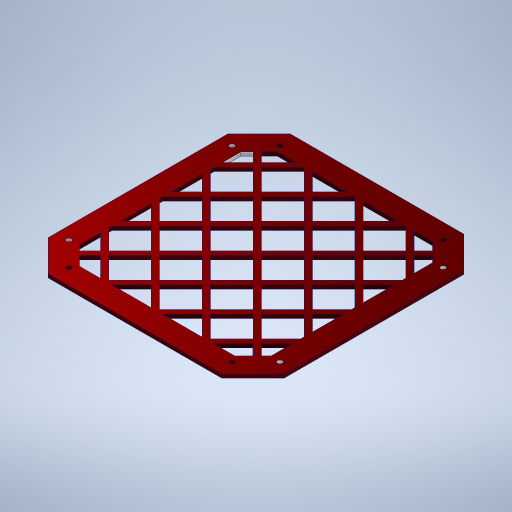
# Autodesk Inventor part: Part2
Saved by Autodesk Inventor 2024.2 (Build 282272000, 272)
## iProperties
Created: 2024-01-05
Part Number: Part2
Material: Aluminum 6061
Document SubType Name: Modeling
Designer: rohan
Density: 2.7 g/cm^3
Appearance: Aluminum - Flat
Author: rohan
Autodesk Inventor part; units mm, degrees
ref_plane "YZ Plane" through (0, 0, 0) normal (1, 0, 0) x (0, 1, 0)
ref_plane "XZ Plane" through (0, 0, 0) normal (0, 1, 0) x (-1, 0, 0)
ref_plane "XY Plane" through (0, 0, 0) normal (0, 0, 1) x (1, 0, 0)
sketch "Sketch4" plane through (0, 0, 0) normal (0, 1, 0) x (-1, 0, 0)
  line L0 (101.6, 104.2289) -> (-101.6, 104.2289)
  line L1 (-101.6, 104.2289) -> (-101.6, -104.2289)
  line L2 (-101.6, -104.2289) -> (101.6, -104.2289)
  line L3 (101.6, -104.2289) -> (101.6, 104.2289)
  line L4 (101.6, 104.2289) -> (-101.6, -104.2289) construction
  line L5 (-101.6, 104.2289) -> (101.6, -104.2289) construction
  point P0 (0, 0)
  dimension "d27" = 203.2
  dimension "d28" = 208.4578
  constraints: 12 end point, 2 midpoint, 2 parallel, 1 horizontal, 1 perpendicular
  measures "d27" distance of L2.end L1.end
  measures "d28" distance of L1.end L0.end
extrude "Extrusion4" add sketch "Sketch4" along normal blind 3.175
sketch "Sketch5" plane through (0, 3.175, 0) normal (0, 1, 0) x (1, 0, 0)
  line L0 (101.6, -104.2289) -> (101.6, 104.2289) projected
  line L1 (101.6, 104.2289) -> (-101.6, 104.2289) projected
  line L2 (-101.6, 104.2289) -> (-101.6, -104.2289) projected
  line L3 (-101.6, -104.2289) -> (101.6, -104.2289) projected
  line L4 (70.2691, 90.8431) -> (-70.2691, 90.8431)
  line L5 (-70.2691, 90.8431) -> (-70.2691, -90.8431)
  line L6 (-70.2691, -90.8431) -> (70.2691, -90.8431)
  line L7 (70.2691, -90.8431) -> (70.2691, 90.8431)
  line L8 (70.2691, 90.8431) -> (-70.2691, -90.8431) construction
  line L9 (-70.2691, 90.8431) -> (70.2691, -90.8431) construction
  circle A0 centre (-70.2691, -90.8431) radius 1.9939
  circle A1 centre (-70.2691, 90.8431) radius 1.9939
  circle A2 centre (70.2691, 90.8431) radius 1.9939
  circle A3 centre (70.2691, -90.8431) radius 1.9939
  point P0 (0, 0)
  dimension "d31" = 203.2
  dimension "d32" = 208.4578
  dimension "d33" = 140.5382
  dimension "d34" = 181.6862
  dimension "d39" = 3.9878
  dimension "d40" = 3.9878
  dimension "d41" = 3.9878
  dimension "d42" = 3.9878
  constraints: 12 end point, 4 centre point, 4 coincident, 2 midpoint, 2 parallel, 1 horizontal, 1 perpendicular
  measures "d31" distance of L2.end L0.start
  measures "d32" distance of L1.end L2.end
  measures "d33" distance of L6.end L5.end
  measures "d34" distance of L5.end L4.end
  measures "d39" diameter of A0
  measures "d40" diameter of A1
  measures "d41" diameter of A2
  measures "d42" diameter of A3
extrude "Extrusion7" cut sketch "Sketch5" against normal blind 26.9875 contours A1 L5 L4 | L4 L5 A1 | A2 L7 L4 | L4 L7 A2 | A0 L6 L5 | L5 L6 A0 | A3 L6 L7 | L7 L6 A3
chamfer "Chamfer1" distance 26.9875 angle 45 1 edges at (101.6, 1.5875, 104.2289)
chamfer "Chamfer2" distance 26.9875 angle 45 3 edges at (101.6, 1.5875, -104.2289) (-101.6, 1.5875, -104.2289) (-101.6, 1.5875, 104.2289)
sketch "Sketch8" plane through (0, 3.175, 0) normal (0, 1, 0) x (1, 0, 0)
  circle A0 centre (70.2691, 90.8431) radius 1.9939 projected
  circle A1 centre (70.2691, -90.8431) radius 1.9939 projected
  circle A2 centre (-70.2691, 90.8431) radius 1.9939 projected
  circle A3 centre (-70.2691, -90.8431) radius 1.9939 projected
  line L0 (-74.6125, -104.2289) -> (-101.6, -77.2414) projected
  line L1 (-74.6125, -104.2289) -> (74.6125, -104.2289) projected
  line L2 (101.6, -77.2414) -> (74.6125, -104.2289) projected
  line L3 (101.6, -77.2414) -> (101.6, 77.2414) projected
  line L4 (74.6125, 104.2289) -> (101.6, 77.2414) projected
  line L5 (74.6125, 104.2289) -> (-74.6125, 104.2289) projected
  line L6 (-101.6, 77.2414) -> (-74.6125, 104.2289) projected
  line L7 (-101.6, 77.2414) -> (-101.6, -77.2414) projected
  line L8 (66.7217, -85.1789) -> (-66.7217, -85.1789)
  line L9 (-66.7217, -85.1789) -> (-82.55, -69.3506)
  line L10 (-82.55, -69.3506) -> (-82.55, 69.3506)
  line L11 (-82.55, 69.3506) -> (-66.7217, 85.1789)
  line L12 (-66.7217, 85.1789) -> (66.7217, 85.1789)
  line L13 (66.7217, 85.1789) -> (82.55, 69.3506)
  line L14 (82.55, 69.3506) -> (82.55, -69.3506)
  line L15 (82.55, -69.3506) -> (66.7217, -85.1789)
  line L16 (82.55, -51.3901) -> (48.7612, -85.1789)
  line L17 (91.8895, -34.8664) -> (32.2375, -94.5184)
  line L18 (85.1946, -41.5613) -> (82.55, -44.2059)
  line L19 (34.1074, -92.6485) -> (41.577, -85.1789)
  line L20 (74.6359, -77.2648) -> (62.9721, -65.601)
  line L21 (69.9776, -12.9546) -> (10.3257, -72.6065)
  line L22 (60.6382, -29.4783) -> (26.8494, -63.2671)
  line L23 (12.1956, -70.7367) -> (19.6652, -63.2671)
  line L24 (63.2827, -19.6495) -> (60.6382, -22.2941)
  line L25 (48.0658, 8.9572) -> (-11.5861, -50.6947)
  line L26 (38.7264, -7.5665) -> (4.9376, -41.3553)
  line L27 (-9.7162, -48.8249) -> (-2.2466, -41.3553)
  line L28 (41.3709, 2.2623) -> (38.7264, -0.3823)
  line L29 (26.154, 30.869) -> (-33.4979, -28.7829)
  line L30 (16.8145, 14.3454) -> (-16.9743, -19.4434)
  line L31 (-31.6281, -26.913) -> (-24.1585, -19.4434)
  line L32 (19.4591, 24.1741) -> (16.8145, 21.5296)
  line L33 (4.2422, 52.7809) -> (-55.4098, -6.8711)
  line L34 (-5.0973, 36.2572) -> (-38.8861, 2.4684)
  line L35 (-53.5399, -5.0012) -> (-46.0703, 2.4684)
  line L36 (-2.4527, 46.086) -> (-5.0973, 43.4414)
  line L37 (-17.6697, 74.6927) -> (-77.3216, 15.0408)
  line L38 (-27.0091, 58.169) -> (-60.7979, 24.3802)
  line L39 (-75.4517, 16.9106) -> (-67.9821, 24.3802)
  line L40 (-24.3646, 67.9978) -> (-27.0091, 65.3532)
  line L41 (-39.5815, 96.6045) -> (-99.2334, 36.9526)
  line L42 (-48.9209, 80.0808) -> (-82.7097, 46.292)
  line L43 (-97.3635, 38.8224) -> (-89.8939, 46.292)
  line L44 (-46.2764, 89.9096) -> (-48.9209, 87.265)
  line L45 (57.2375, -32.8789) -> (82.55, -7.5665)
  line L46 (57.2375, -25.6947) -> (85.4007, 2.4684)
  line L47 (23.2573, -59.675) -> (-7.8029, -90.7352)
  line L48 (30.4415, -59.675) -> (-0.6187, -90.7352)
  line L49 (-5.9814, -45.0901) -> (-51.6265, -90.7352)
  line L50 (8.5297, -37.7631) -> (-46.2764, -92.5692)
  line L51 (33.3382, -12.9546) -> (85.4007, 39.1078)
  line L52 (38.7264, -0.3823) -> (91.8895, 52.7809)
  line L53 (8.5297, 6.0605) -> (79.7339, 77.2648)
  line L54 (8.5297, 13.2447) -> (79.7339, 84.449)
  line L55 (-10.4855, -12.9546) -> (-77.3216, -79.7907)
  line L56 (-24.9377, -20.2227) -> (-82.7097, -77.9947)
  line L57 (-32.3973, 8.9572) -> (-97.3635, -56.0091)
  line L58 (-43.9035, 4.6352) -> (-89.8939, -41.3553)
  line L59 (-15.1552, 26.1993) -> (48.5551, 89.9096)
  line L60 (-15.1552, 33.3835) -> (41.3709, 89.9096)
  line L61 (-37.067, 48.1111) -> (4.7315, 89.9096)
  line L62 (-34.3079, 58.0544) -> (4.2422, 96.6045)
  line L63 (-66.163, 26.1993) -> (-92.7446, -0.3823)
  line L64 (-51.7946, 33.3835) -> (-96.7913, -11.6132)
  line L65 (0, -118.764) -> (0, 117.8885)
  line L66 (-82.55, -51.3901) -> (-48.7612, -85.1789)
  line L67 (-91.8895, -34.8664) -> (-32.2375, -94.5184)
  line L68 (-69.9776, -12.9546) -> (-10.3257, -72.6065)
  line L69 (-60.6382, -29.4783) -> (-26.8494, -63.2671)
  line L70 (-48.0658, 8.9572) -> (11.5861, -50.6947)
  line L71 (-38.7264, -7.5665) -> (-4.9376, -41.3553)
  line L72 (9.7162, -48.8249) -> (2.2466, -41.3553)
  line L73 (-26.154, 30.869) -> (33.4979, -28.7829)
  line L74 (-16.8145, 14.3454) -> (16.9743, -19.4434)
  line L75 (31.6281, -26.913) -> (24.1585, -19.4434)
  line L76 (-19.4591, 24.1741) -> (-16.8145, 21.5296)
  line L77 (-4.2422, 52.7809) -> (55.4098, -6.8711)
  line L78 (5.0973, 36.2572) -> (38.8861, 2.4684)
  line L79 (53.5399, -5.0012) -> (46.0703, 2.4684)
  line L80 (2.4527, 46.086) -> (5.0973, 43.4414)
  line L81 (17.6697, 74.6927) -> (77.3216, 15.0408)
  line L82 (27.0091, 58.169) -> (60.7979, 24.3802)
  line L83 (75.4517, 16.9106) -> (67.9821, 24.3802)
  line L84 (24.3646, 67.9978) -> (27.0091, 65.3532)
  line L85 (39.5815, 96.6045) -> (99.2334, 36.9526)
  line L86 (48.9209, 80.0808) -> (82.7097, 46.292)
  line L87 (-57.2375, -32.8789) -> (-82.55, -7.5665)
  line L88 (-57.2375, -25.6947) -> (-85.4007, 2.4684)
  line L89 (-23.2573, -59.675) -> (7.8029, -90.7352)
  line L90 (-30.4415, -59.675) -> (0.6187, -90.7352)
  line L91 (5.9814, -45.0901) -> (51.6265, -90.7352)
  line L92 (-8.5297, -37.7631) -> (46.2764, -92.5692)
  line L93 (-33.3382, -12.9546) -> (-85.4007, 39.1078)
  line L94 (-38.7264, -0.3823) -> (-91.8895, 52.7809)
  line L95 (-8.5297, 6.0605) -> (-79.7339, 77.2648)
  line L96 (-8.5297, 13.2447) -> (-79.7339, 84.449)
  line L97 (10.4855, -12.9546) -> (77.3216, -79.7907)
  line L98 (24.9377, -20.2227) -> (82.7097, -77.9947)
  line L99 (32.3973, 8.9572) -> (97.3635, -56.0091)
  line L100 (43.9035, 4.6352) -> (89.8939, -41.3553)
  line L101 (15.1552, 26.1993) -> (-48.5551, 89.9096)
  line L102 (15.1552, 33.3835) -> (-41.3709, 89.9096)
  line L103 (37.067, 48.1111) -> (-4.7315, 89.9096)
  line L104 (34.3079, 58.0544) -> (-4.2422, 96.6045)
  line L105 (66.163, 26.1993) -> (92.7446, -0.3823)
  line L106 (51.7946, 33.3835) -> (96.7913, -11.6132)
  line L107 (57.2058, 71.796) -> (43.8244, 85.1789)
  line L108 (-51.6723, 77.3295) -> (-41.3709, 87.6309)
  point P0 (0, 0)
  point P1 (-62.9721, -65.601)
  point P2 (-18.3197, -64.6125)
  point P3 (0, -82.9323)
  point P4 (18.3197, -64.6125)
  point P5 (0, -46.2928)
  point P6 (-4.9376, -85.1789)
  point P7 (-21.9118, -68.2046)
  point P8 (-38.8861, -85.1789)
  point P9 (38.8861, -85.1789)
  point P10 (21.9118, -68.2046)
  point P11 (4.9376, -85.1789)
  point P12 (69.3276, -20.7889)
  point P13 (82.55, -34.0113)
  point P14 (65.6556, -68.2845)
  point P15 (69.3276, -64.6125)
  point P16 (78.3078, -73.5928)
  point P17 (82.55, -41.1955)
  point P18 (65.7355, -24.381)
  point P19 (47.4158, -42.7007)
  point P20 (65.7355, -61.0204)
  point P21 (25.5039, -64.6125)
  point P22 (43.8236, -82.9323)
  point P23 (62.1434, -64.6125)
  point P24 (43.8236, -46.2928)
  point P25 (21.9118, -61.0204)
  point P26 (40.2315, -42.7007)
  point P27 (21.9118, -24.381)
  point P28 (3.5921, -42.7007)
  point P29 (62.1434, -20.7889)
  point P30 (43.8236, -2.4692)
  point P31 (25.5039, -20.7889)
  point P32 (43.8236, -39.1086)
  point P33 (82.55, 2.6281)
  point P34 (65.7355, 19.4427)
  point P35 (47.4158, 1.1229)
  point P36 (65.7355, -17.1968)
  point P37 (82.55, -0.3823)
  point P38 (82.55, 9.8123)
  point P39 (82.55, 36.2572)
  point P40 (69.3276, 23.0348)
  point P41 (0, -2.4692)
  point P42 (-18.3197, -20.7889)
  point P43 (0, -39.1086)
  point P44 (18.3197, -20.7889)
  point P45 (-69.3276, 23.0348)
  point P46 (-82.55, 36.2572)
  point P47 (-82.55, 9.8123)
  point P48 (-69.3276, -20.7889)
  point P49 (-82.55, -34.0113)
  point P50 (-65.7355, -24.381)
  point P51 (-82.55, -41.1955)
  point P52 (-82.55, -44.2059)
  point P53 (-65.7355, -61.0204)
  point P54 (-47.4158, -42.7007)
  point P55 (-69.3276, -64.6125)
  point P56 (-78.3078, -73.5928)
  point P57 (-65.7355, -68.2046)
  point P58 (-74.7157, -77.1849)
  point P59 (-43.8236, -46.2928)
  point P60 (-62.1434, -64.6125)
  point P61 (-43.8236, -82.9323)
  point P62 (-25.5039, -64.6125)
  point P63 (-21.9118, -24.381)
  point P64 (-40.2315, -42.7007)
  point P65 (-21.9118, -61.0204)
  point P66 (-11.5861, -50.6947)
  point P67 (-3.5921, -42.7007)
  point P68 (21.9118, 19.4427)
  point P69 (3.5921, 1.1229)
  point P70 (21.9118, -17.1968)
  point P71 (40.2315, 1.1229)
  point P72 (0, 4.715)
  point P73 (18.3197, 23.0348)
  point P74 (0, 41.3545)
  point P75 (-18.3197, 23.0348)
  point P76 (-40.2315, 1.1229)
  point P77 (-21.9118, -17.1968)
  point P78 (-3.5921, 1.1229)
  point P79 (-21.9118, 19.4427)
  point P80 (-43.8236, -2.4692)
  point P81 (-62.1434, -20.7889)
  point P82 (-43.8236, -39.1086)
  point P83 (-33.4979, -28.7829)
  point P84 (-25.5039, -20.7889)
  point P85 (-47.4158, 1.1229)
  point P86 (-65.7355, 19.4427)
  point P87 (-82.55, 2.6281)
  point P88 (-82.55, -0.3823)
  point P89 (-65.7355, -17.1968)
  point P90 (-62.1434, 23.0348)
  point P91 (-43.8236, 4.715)
  point P92 (-25.5039, 23.0348)
  point P93 (-43.8236, 41.3545)
  point P94 (-3.5921, 44.9466)
  point P95 (-21.9118, 63.2663)
  point P96 (-40.2315, 44.9466)
  point P97 (-21.9118, 26.6269)
  point P98 (-73.5928, 78.3078)
  point P99 (-65.7355, 70.4505)
  point P100 (-51.0071, 85.1789)
  point P101 (-82.55, 43.4414)
  point P102 (-65.7355, 26.6269)
  point P103 (-47.4158, 44.9466)
  point P104 (-65.7355, 63.2663)
  point P105 (-82.55, 46.4518)
  point P106 (-43.8236, 85.1781)
  point P107 (-62.1434, 66.8584)
  point P108 (-43.8236, 48.5387)
  point P109 (-25.5039, 66.8584)
  point P110 (-36.6402, 85.1789)
  point P111 (-21.9118, 70.4505)
  point P112 (-7.1834, 85.1789)
  point P113 (0, 48.5387)
  point P114 (18.3197, 66.8584)
  point P115 (0, 85.1781)
  point P116 (-18.3197, 66.8584)
  point P117 (40.2315, 44.9466)
  point P118 (21.9118, 63.2663)
  point P119 (3.5921, 44.9466)
  point P120 (21.9118, 26.6269)
  point P121 (43.8236, 41.3545)
  point P122 (25.5039, 23.0348)
  point P123 (43.8236, 4.715)
  point P124 (62.1434, 23.0348)
  point P125 (47.4158, 44.9466)
  point P126 (65.7355, 26.6269)
  point P127 (82.55, 43.4414)
  point P128 (82.55, 46.4518)
  point P129 (65.7355, 63.2663)
  point P130 (69.3276, 66.8584)
  point P131 (82.55, 53.636)
  point P132 (77.1849, 74.7157)
  point P133 (51.0071, 85.1789)
  point P134 (65.7355, 70.4505)
  point P135 (73.5928, 78.3078)
  point P136 (25.5039, 66.8584)
  point P137 (43.8236, 48.5387)
  point P138 (62.1434, 66.8584)
  point P139 (21.9118, 70.4505)
  point P140 (36.6402, 85.1789)
  point P141 (7.1834, 85.1789)
  point P142 (-69.3276, 66.8584)
  point P143 (-77.1849, 74.7157)
  point P144 (-82.55, 53.636)
  dimension "d51" = 19.05
  dimension "d52" = 12.7
  dimension "d53" = 5.08
  dimension "d56" = 30.988
  constraints: 202 end point, 100 point on line, 83 symmetric about line, 5 parallel, 2 midpoint, 2 perpendicular, 1 vertical, 80 other
  measures "d51" distance between parallel lines of L2 L15
  measures "d52" distance between parallel lines of L16 L15
  measures "d53" distance between parallel lines of L16 L17
  measures "d56" distance of L19.start L23.start
extrude "Extrusion8" cut sketch "Sketch8" against normal blind 9.525 contours L48 L92 L8 | L65 L92 L21 L47 | L89 L68 L50 L65 | L8 L50 L90 | L65 L77 L102 L61 | L103 L60 L33 L65 | L48 L22 L97 L17 L91 | L50 L26 L97 L21 L91 L70 | L65 L74 L97 L25 | L70 L55 L30 L65 | L25 L49 L68 L55 L71 L92 | L49 L67 L55 L69 L90 | L62 L37 L102 L12 | L12 L60 L81 L104 | L101 L33 L73 L96 L38 L61 | L65 L73 L34 L59 | L101 L78 L29 L65 | L103 L82 L54 L29 L77 L59 | L16 L20 L15 L8 | L73 L30 L53 L78 L99 L25 | L29 L70 L57 L34 L95 L74 | L8 L9 L55 L66 | L101 L37 L96 L42 L108 | L107 L86 L54 L81 L59 | L98 L22 L45 L99 L14 L17 | L26 L51 L99 L21 L98 L73 | L29 L56 L68 L57 L93 L71 | L67 L10 L57 L87 L69 L56 | L41 L96 L11 L12 | L12 L13 L54 L85 | L16 L14 L15 L98 | L56 L9 L10 L66 | L70 L94 L64 L38 L95 L33 | L41 L10 L11 L95 | L53 L13 L14 L85 | L82 L106 L52 L25 L77 L53 | L100 L45 L14 | L51 L106 L14 L46 L21 L100 L77 | L33 L58 L68 L88 L10 L64 L93 | L10 L87 L58 | L95 L37 L94 L10 L42 | L86 L14 L52 L81 L53 | L51 L14 L105 L81 | L37 L63 L10 L93
sketch "Sketch9" plane through (0, 3.175, 0) normal (0, 1, 0) x (1, 0, 0)
  circle A0 centre (70.2691, -90.8431) radius 1.9939 projected
  circle A1 centre (-70.2691, 90.8431) radius 1.9939 projected
  line L0 (70.2691, -90.8431) -> (-70.2691, -90.8431)
  line L1 (-70.2691, -90.8431) -> (-70.2691, 90.8431)
  line L2 (-70.2691, 90.8431) -> (70.2691, 90.8431)
  line L3 (70.2691, 90.8431) -> (70.2691, -90.8431)
  line L4 (90.8431, 70.2691) -> (-90.8431, 70.2691)
  line L5 (-90.8431, 70.2691) -> (-90.8431, -70.2691)
  line L6 (-90.8431, -70.2691) -> (90.8431, -70.2691)
  line L7 (90.8431, -70.2691) -> (90.8431, 70.2691)
  line L8 (90.8431, 70.2691) -> (-90.8431, -70.2691) construction
  line L9 (-90.8431, 70.2691) -> (90.8431, -70.2691) construction
  circle A2 centre (90.8431, -70.2691) radius 1.9939
  circle A3 centre (-90.8431, -70.2691) radius 1.9939
  circle A4 centre (90.8431, 70.2691) radius 1.9939
  circle A5 centre (-90.8431, 70.2691) radius 1.9939
  point P0 (0, 0)
  dimension "d63" = 181.6862
  dimension "d64" = 140.5382
  dimension "d65" = 181.6862
  dimension "d66" = 140.5382
  dimension "d67" = 3.9878
  dimension "d68" = 3.9878
  dimension "d69" = 3.9878
  dimension "d70" = 3.9878
  constraints: 20 end point, 4 centre point, 4 coincident, 4 parallel, 2 horizontal, 2 midpoint, 2 perpendicular
  measures "d63" distance of L0.end L1.end
  measures "d64" distance of L0.start L0.end
  measures "d65" distance of L6.end L5.end
  measures "d66" distance of L5.end L4.end
  measures "d67" diameter of A2
  measures "d68" diameter of A3
  measures "d69" diameter of A4
  measures "d70" diameter of A5
extrude "Extrusion9" cut sketch "Sketch9" against normal blind 31.75 contours A2 L7 L6 | L6 L7 A2 | A4 L7 L4 | L4 L7 A4 | A3 L5 L6 | L6 L5 A3 | A5 L5 L4 | L4 L5 A5
body "Solid2"
